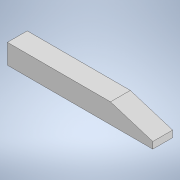
# Autodesk Inventor part: Garra2
Saved by Autodesk Inventor 2021 (Build 250183000, 183)
## iProperties
Created: 2022-02-15
Part Number: Garra2
Material: Genérico
Document SubType Name: Modeling
Designer: aluno
Density: 1 g/cm^3
Appearance: Padrão
Author: aluno
Autodesk Inventor part; units mm, degrees
ref_plane "YZ Plane" through (0, 0, 0) normal (1, 0, 0) x (0, 1, 0)
ref_plane "XZ Plane" through (0, 0, 0) normal (0, 1, 0) x (-1, 0, 0)
ref_plane "XY Plane" through (0, 0, 0) normal (0, 0, 1) x (1, 0, 0)
sketch "Esboço1" plane through (0, 0, 0) normal (0, 0, 1) x (1, 0, 0)
  line L0 (0, 0) -> (110, 0)
  line L1 (110, 0) -> (110, 15)
  line L2 (110, 15) -> (0, 15)
  line L3 (0, 15) -> (0, 0)
  dimension "d0" = 110
  dimension "d1" = 15
  constraints: 8 end point, 2 parallel, 1 horizontal, 1 perpendicular
  measures "d0" distance of L2.end L1.end
  measures "d1" distance of L1.end L0.end
extrude "Extrusão1" add sketch "Esboço1" along normal blind 15
chamfer "Chanfro1" distance 10 distance2 32 1 edges at (110, 15, 7.5) measured on face at (110, 14.5, 7.5)
sketch "Esboço2" plane through (0, 0, 0) normal (0, -1, 0) x (1, 0, 0)
  line L0 (0, 15) -> (110, 15) projected
  line L1 (0, 0) -> (0, 15) projected
  point P0 (13, 7.5)
  point P1 (66, 7.5)
  dimension "d7" = 7.5
  dimension "d8" = 13
  dimension "d25" = 53
  constraints: 1 horizontal alignment
  measures "d7" distance from line of L0 point (13, 7.5)
  measures "d8" distance from line of L1 point (13, 7.5)
  measures "d25" distance of point (66, 7.5) point (13, 7.5)
hole "Furo1" at (13, 0, 7.5) direction (0, 1, 0) diameter 8 depth 10.4 tip angle 118
